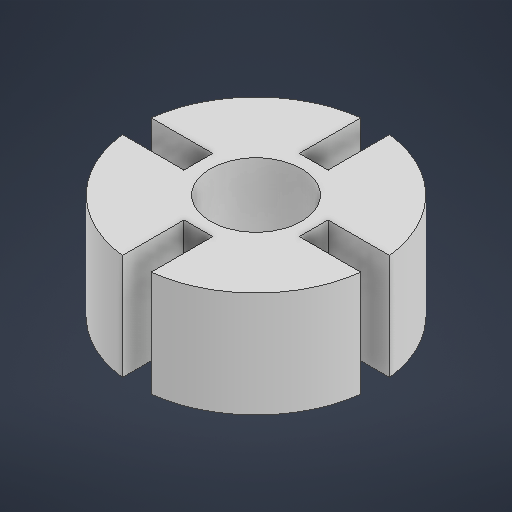
# Autodesk Inventor part: rotor
Saved by Autodesk Inventor 2025.3 (Build 293356000, 356)
## iProperties
Created: 2025-10-20
Part Number: rotor
Material: Generic
Document SubType Name: Modeling
Designer: sophi
Density: 1 g/cm^3
Appearance: Default
Author: sophi
Autodesk Inventor part; units mm, degrees
ref_plane "YZ Plane" through (0, 0, 0) normal (1, 0, 0) x (0, 1, 0)
ref_plane "XZ Plane" through (0, 0, 0) normal (0, 1, 0) x (-1, 0, 0)
ref_plane "XY Plane" through (0, 0, 0) normal (0, 0, 1) x (1, 0, 0)
sketch "Sketch1" plane through (0, 0, 0) normal (0, 1, 0) x (-1, 0, 0)
  circle A0 centre (0, 0) radius 25
  line L0 (27, 3) -> (12, 3)
  line L1 (12, 3) -> (12, -3)
  line L2 (12, -3) -> (27, -3)
  line L3 (27, -3) -> (27, 3)
  line L4 (0, 35.0975) -> (0, -33.454) construction
  line L5 (19.7931, 0) -> (-19.2285, 0) construction
  circle A1 centre (0, 0) radius 9.5
  line L6 (-3, 27) -> (-3, 12)
  line L7 (3, 12) -> (3, 27)
  line L8 (-3, 12) -> (3, 12)
  line L9 (-27, -3) -> (-12, -3)
  line L10 (-12, 3) -> (-27, 3)
  line L11 (-12, -3) -> (-12, 3)
  line L12 (3, -27) -> (3, -12)
  line L13 (-3, -12) -> (-3, -27)
  line L14 (3, -12) -> (-3, -12)
  point P0 (24.8193, 3)
  point P1 (3, 24.8193)
  point P2 (-3, 24.8193)
  point P3 (-24.8193, 3)
  point P4 (-24.8193, -3)
  point P5 (-3, -24.8193)
  point P6 (3, -24.8193)
  point P7 (24.8193, -3)
  dimension "d0" = 50
  dimension "d1" = 6
  dimension "d3" = 19
  dimension "d4" = 12
  dimension "d5" = 15
  dimension "d8" = 360
  constraints: 30 end point, 2 centre point, 2 coincident, 2 horizontal, 2 parallel, 2 point on line, 1 perpendicular, 1 vertical, 30 other
  measures "d0" diameter of A0
  measures "d1" distance of L2.end L0.start
  measures "d3" diameter of A1
  measures "d4" distance from line of point (0, 0) L1
  measures "d5" distance of L1.end L2.end
extrude "Extrusion1" add sketch "Sketch1" along normal blind 22 contours L0 L1 L2 A0 L12 L14 L13 L9 L11 L10 L6 L8 L7
body "Solid1"
